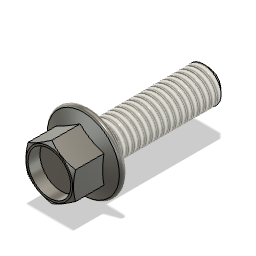
Motor_Mount v1 (Autodesk Fusion 360 archive; units mm, degrees)
design "Indented Hex Flange Head Machine Screw ANSI B18.6.7M - M6x1 x 20 Steel Grade 2 Plain"
description: Indented Hex Flange Head Machine Screw ANSI B18.6.7M - M6x1 x 20
Autodesk Fusion 360 part; units mm, degrees
sketch "Sketch1" plane through (0, 0, 0) normal (0, 1, 0) x (1, 0, 0)
  line L0 (-3, 0) -> (-3, 20)
  line L1 (-3, 20) -> (0, 20)
  line L2 (0, 20) -> (0, -4.7)
  line L3 (-3, 0) -> (-4.62, 0)
  line L4 (-4.62, 0) -> (-4.62, -6.2959)
  line L5 (-3.92, -6.7) -> (-3.6, -6.7)
  line L6 (-3.92, -6.7) -> (-4.62, -6.2959)
  line L7 (-3.6, -6.7) -> (-3.6, -4.7)
  line L8 (-3.6, -4.7) -> (0, -4.7)
  dimension "d9" = 6
  dimension "d68" = 20
  dimension "d111" = 6.7
  dimension "d113" = 30
  dimension "d114" = 9.24
  dimension "d115" = 7.84
  dimension "d158" = 7.2
  dimension "d159" = 2
  constraint perpendicular L0 L1
  constraint perpendicular L0 L3
  constraint coincident origin L3
  constraint vertical L0
  constraint vertical L2
  constraint parallel L2 L4
  constraint coincident L2 L8.end
  constraint perpendicular L2 L5
  constraint coincident L3.end L4.start
  constraint perpendicular L5 L7
  constraint perpendicular L2 L8
  constraint coincident L2.end L8.end
  constraint coincident origin L2
  measures "d68" distance of origin L1.end
  measures "d111" distance of L3 L5
  measures "d113" angle of L5 L6
  measures "d159" distance of L5.end L7.end
revolve "Revolve1" add sketch "Sketch1" angle 360 about axis through (0, 0, -20) along (0, 0, 1)
sketch "Sketch8" plane through (0, 0, 0) normal (0, 0, 1) x (1, 0, 0)
  line L0 (0, 0) -> (-4, 0) construction
  line L1 (-4, -2.3118) -> (-4, 2.3118)
  circle A0 centre (0, 0) radius 4.62
  dimension "d110" = 4
  constraint horizontal L0
  constraint perpendicular L0 L1
  constraint coincident L0.end L1
  constraint coincident L0.start A0.centre
  constraint coincident L1.end A0
  constraint coincident L1.start A0
  measures "d110" distance of L0.start L1
extrude "Extrude5" cut sketch "Sketch8" along normal blind 6.7 contours L1 A0 picked at (-4.1, -0.5631)
pattern_circular "C-Pattern2" count 6 over 360 about axis through (0, 0, 1.75) along (0, 0, 1) of "Extrude5"
sketch "Sketch12" plane through (0, 0, 0) normal (0, 1, 0) x (1, 0, 0)
  line L0 (3.8, 0) -> (5.8845, 0)
  line L1 (6.0608, -1) -> (3.8, -1.8229)
  line L2 (3.8, -1.8229) -> (3.8, 0)
  arc A0 (6.0608, -1) -> (5.8845, 0) centre (5.8845, -0.5155) ccw
  line L3 (0, -1.75) -> (0, -22.5)
  line L4 (4.62, 0) -> (4.62, -1.5244) construction
  line L5 (0, 0) -> (4, 0)
  line L6 (6.4, 0) -> (6.4, -1.8229) construction
  line L7 (3.8, -1.8229) -> (6.4, -1.8229) construction
  dimension "d122" = 7.6
  dimension "d126" = 9.24
  dimension "d138" = 1
  dimension "d142" = 6.4
  dimension "d163" = 20
  constraint horizontal L0
  constraint perpendicular L0 L2
  constraint tangent L0 A0
  constraint tangent L1 A0
  constraint horizontal L5.start L0.start
  constraint coincident L1 L4.end
  constraint perpendicular L0 L4
  constraint coincident L0 L4.start
  constraint vertical L6
  constraint tangent A0 L6
  constraint coincident L0 L6.start
  constraint perpendicular L6 L7
  constraint coincident L6.end L7.end
  measures "d138" vertical distance of L0.end L1.start
  measures "d142" distance of L5.start L6
  measures "d163" angle of L0 L1
revolve "Revolve3" add sketch "Sketch12" angle 360 about axis through (0, 0, 1.75) along (0, 0, 1)
thread "Thread2" "ISO Metric profile 6.0 M6x1 6g" major diameter 5.884 minor diameter 4.7435 pitch 1 angle 60 resizes the face on face at (-2.9851, 0.2987, -6.6667) from (0, 0, -2.3) to (0, 0, -20)
fillet "Fillet4" radius 0.2 1 edges at (2.7429, -1.0639, 0)
sketch "Sketch5" plane through (0, 0, 0) normal (0, 1, 0) x (1, 0, 0)
  line L0 (-3.06, 19.125) -> (-2.125, 20)
  line L1 (0, -1.75) -> (0, -22.5)
  line L2 (0, 20) -> (0, -4.7)
  line L3 (0, 20) -> (-3.06, 20)
  line L4 (-3.06, 20) -> (-3.06, 19.125)
  dimension "d153" = 2.125
  dimension "d156" = 3.06
  dimension "d157" = 0.875
  constraint coincident L2.start L3.start
  constraint perpendicular L2 L3
  constraint coincident L0.end L3
  constraint perpendicular L3 L4
  measures "d153" distance of L0.end L1
  measures "d156" horizontal distance of origin L3.end
  measures "d157" distance of L0.start L3.end
revolve "Revolve2" cut sketch "Sketch5" angle 360 about axis through (0, 0, -20) along (0, 0, 1)
equation "d9 = adsk_nomdia"
equation "adsk_nomlen = 20.00 mm"
equation "adsk_headh = 6.70 mm"
equation "adsk_nomdia = 6.00 mm"
equation "d68 = adsk_nomlen"
equation "d89 = adsk_headh"
equation "adsk_waflat = 8.00 mm"
equation "d110 = adsk_waflat / 2"
equation "d111 = adsk_headh"
equation "d113 = adsk_chamang2"
equation "d114 = adsk_wacor"
equation "d115 = adsk_topdia"
equation "d122 = adsk_waflat * 0.95"
equation "d126 = adsk_waflat * 1.155"
equation "adsk_headdia = 12.80 mm"
equation "adsk_flngheig = 1.00 mm"
equation "adsk_thrlen = 17.70 mm"
equation "d133 = adsk_nomdia / 30"
equation "d138 = adsk_flngheig"
equation "d142 = adsk_headdia / 2"
equation "d144 = adsk_thrlen"
equation "adsk_endpointdia = 4.25 mm"
equation "d153 = adsk_endpointdia / 2"
equation "adsk_startlen = 0.875 mm"
equation "d156 = adsk_nomdia * 0.51"
equation "d157 = adsk_startlen"
equation "d158 = adsk_indentdia"
equation "d159 = adsk_indentdepth"
equation "adsk_wacor = 9.24 mm"
equation "adsk_topdia = adsk_waflat * 0.98"
equation "adsk_chamang2 = 30.00 deg"
equation "d163 = adsk_flngang"
equation "adsk_flngang = 20.00 deg"
equation "adsk_indentdia = 7.20 mm"
equation "adsk_indentdepth = 2.00 mm"
